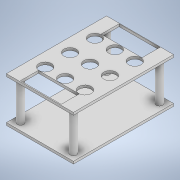
# Autodesk Inventor part: Elve tube holder
Saved by Autodesk Inventor 2020 (Build 240168000, 168)
## iProperties
Created: 2022-03-03
Part Number: Elve tube holder
Material: Generic
Document SubType Name: Modeling
Designer: Beaucage
Density: 1 g/cm^3
Appearance: Default
Author: Beaucage
Autodesk Inventor part; units mm, degrees
ref_plane "YZ Plane" through (0, 0, 0) normal (1, 0, 0) x (0, 1, 0)
ref_plane "XZ Plane" through (0, 0, 0) normal (0, 1, 0) x (-1, 0, 0)
ref_plane "XY Plane" through (0, 0, 0) normal (0, 0, 1) x (1, 0, 0)
sketch "Sketch1" plane through (0, 0, 0) normal (0, 1, 0) x (-1, 0, 0)
  line L0 (0, 0) -> (85.48, 0)
  line L1 (85.48, 0) -> (85.48, -127.76)
  line L2 (85.48, -127.76) -> (0, -127.76)
  line L3 (0, -127.76) -> (0, 0)
  dimension "d0" = 85.48
  dimension "d1" = 127.76
  constraints: 8 end point, 2 parallel, 1 horizontal, 1 perpendicular
  measures "d0" distance of L1.end L2.end
  measures "d1" distance of L0.end L1.end
extrude "Extrusion1" add sketch "Sketch1" along normal blind 3.175
sketch "Sketch2" plane through (0, 3.175, 0) normal (0, 1, 0) x (1, 0, 0)
  line L0 (0, 0) -> (-8.9803, 8.9803)
  line L1 (-85.48, 127.76) -> (-85.48, 0) projected
  line L2 (-85.48, 0) -> (-76.4997, 8.9803)
  line L3 (-85.48, 0) -> (-72.78, 0) construction
  line L4 (0, 127.76) -> (-85.48, 127.76) projected
  line L5 (-85.48, 127.76) -> (-76.4997, 118.7797)
  line L6 (-85.48, 127.76) -> (-72.78, 127.76) construction
  line L7 (0, 127.76) -> (-8.9803, 118.7797)
  circle A0 centre (-76.4997, 118.7797) radius 4.1275
  circle A1 centre (-8.9803, 118.7797) radius 4.1275
  circle A2 centre (-76.4997, 8.9803) radius 4.1275
  circle A3 centre (-8.9803, 8.9803) radius 4.1275
  dimension "d4" = 12.7
  dimension "d5" = 12.7
  dimension "d6" = 45
  dimension "d7" = 12.7
  dimension "d8" = 45
  dimension "d9" = 12.7
  dimension "d10" = 8.255
  dimension "d11" = 8.255
  dimension "d12" = 8.255
  dimension "d13" = 8.255
  constraints: 12 end point, 4 centre point, 4 coincident, 2 equal length, 2 horizontal
  measures "d4" distance of L0.start L0.end
  measures "d5" distance of L1.end L2.end
  measures "d6" angle of L3 L2
  measures "d7" distance of L1.start L5.end
  measures "d8" angle of L5 L6
  measures "d9" distance of L4.start L7.end
  measures "d10" diameter of A0
  measures "d11" diameter of A1
  measures "d12" diameter of A2
  measures "d13" diameter of A3
extrude "Extrusion2" add sketch "Sketch2" along normal blind 50.8
sketch "Sketch3" plane through (-76.4997, 53.975, -8.9803) normal (0, 1, 0) x (1, 0, 0)
  line L0 (-8.9803, -8.9803) -> (76.4997, -8.9803) projected
  line L1 (-8.9803, 118.7797) -> (-8.9803, -8.9803) projected
  line L2 (76.4997, 118.7797) -> (-8.9803, 118.7797) projected
  line L3 (76.4997, -8.9803) -> (76.4997, 118.7797) projected
extrude "Extrusion3" add sketch "Sketch3" along normal blind 3.175
sketch "Sketch4" plane through (-76.4997, 57.15, -8.9803) normal (0, 1, 0) x (1, 0, 0)
  line L0 (-8.9803, -8.9803) -> (76.4997, -8.9803) projected
  line L1 (33.7597, -8.9803) -> (33.7597, 118.7797)
  line L2 (76.4997, 118.7797) -> (-8.9803, 118.7797) projected
  line L3 (33.7597, 54.8997) -> (33.7597, 86.6497)
  line L4 (33.7597, 54.8997) -> (65.5097, 54.8997) construction
  line L5 (33.7597, 54.8997) -> (33.7597, 23.1497)
  circle A0 centre (33.7597, 86.6497) radius 7.874
  circle A1 centre (33.7597, 23.1497) radius 7.874
  circle A2 centre (33.7597, 54.8997) radius 7.874
  line L6 (33.7597, 86.6497) -> (59.1597, 86.6497)
  circle A3 centre (59.1597, 86.6497) radius 7.874
  line L7 (33.7597, 86.6497) -> (8.3597, 86.6497)
  line L8 (33.7597, 54.8997) -> (59.1597, 54.8997)
  line L9 (33.7597, 54.8997) -> (8.3597, 54.8997)
  line L10 (33.7597, 23.1497) -> (59.1597, 23.1497)
  line L11 (33.7597, 23.1497) -> (8.3597, 23.1497)
  line L12 (33.7597, 23.1497) -> (59.1597, 23.1497) construction
  circle A4 centre (8.3597, 86.6497) radius 7.874
  circle A5 centre (8.3597, 54.8997) radius 7.874
  circle A6 centre (59.1597, 54.8997) radius 7.874
  circle A7 centre (59.1597, 23.1497) radius 7.874
  circle A8 centre (8.3597, 23.1497) radius 7.874
  line L13 (7.7247, 95.1761) -> (59.7947, 95.1761)
  line L14 (59.7947, 95.1761) -> (59.7947, 118.0361)
  line L15 (59.7947, 118.0361) -> (7.7247, 118.0361)
  line L16 (7.7247, 118.0361) -> (7.7247, 95.1761)
  line L17 (7.7247, 95.1761) -> (59.7947, 118.0361) construction
  line L18 (59.7947, 95.1761) -> (7.7247, 118.0361) construction
  line L19 (7.7247, 15.1012) -> (59.7947, 15.1012)
  line L20 (59.7947, 15.1012) -> (59.7947, -7.7588)
  line L21 (59.7947, -7.7588) -> (7.7247, -7.7588)
  line L22 (7.7247, -7.7588) -> (7.7247, 15.1012)
  line L23 (7.7247, 15.1012) -> (59.7947, -7.7588) construction
  line L24 (59.7947, 15.1012) -> (7.7247, -7.7588) construction
  point P0 (33.7597, 106.6061)
  point P1 (33.7597, 3.6712)
  dimension "d18" = 31.75
  dimension "d19" = 90
  dimension "d20" = 31.75
  dimension "d21" = 15.748
  dimension "d22" = 15.748
  dimension "d25" = 15.748
  dimension "d26" = 25.4
  dimension "d27" = 15.748
  dimension "d28" = 25.4
  dimension "d29" = 25.4
  dimension "d30" = 25.4
  dimension "d31" = 25.4
  dimension "d32" = 25.4
  dimension "d33" = 180
  dimension "d34" = 15.748
  dimension "d35" = 15.748
  dimension "d36" = 15.748
  dimension "d37" = 15.748
  dimension "d38" = 15.748
  dimension "d39" = 52.07
  dimension "d40" = 22.86
  dimension "d41" = 52.07
  dimension "d42" = 22.86
  constraints: 46 end point, 9 centre point, 9 coincident, 9 horizontal, 7 midpoint, 4 parallel, 4 point on line, 2 equal length, 2 perpendicular, 1 collinear
  measures "d18" distance of L3.start L3.end
  measures "d19" angle of L4 L3
  measures "d20" distance of L3.start L5.end
  measures "d21" diameter of A0
  measures "d22" diameter of A1
  measures "d25" diameter of A2
  measures "d26" distance of L6.start L6.end
  measures "d27" diameter of A3
  measures "d28" distance of L6.start L7.end
  measures "d29" distance of L8.start L8.end
  measures "d30" distance of L8.start L9.end
  measures "d31" distance of L10.start L10.end
  measures "d32" distance of L10.start L11.end
  measures "d33" angle of L11 L12
  measures "d34" diameter of A4
  measures "d35" diameter of A5
  measures "d36" diameter of A6
  measures "d37" diameter of A7
  measures "d38" diameter of A8
  measures "d39" distance of L15.end L14.end
  measures "d40" distance of L14.end L13.end
  measures "d41" distance of L20.end L21.end
  measures "d42" distance of L19.end L20.end
extrude "Extrusion4" cut sketch "Sketch4" against normal blind 3.175
body "Solid1"
